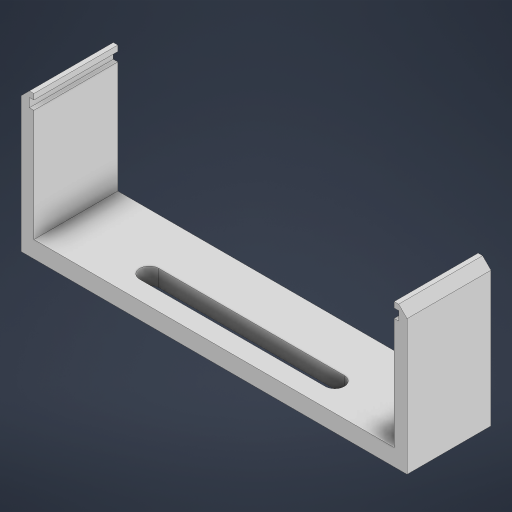
# Autodesk Inventor part: Discovery boar clamp
Saved by Autodesk Inventor 2023 (Build 270158000, 158)
## iProperties
Created: 2024-01-04
Part Number: Discovery boar clamp
Material: Generic
Document SubType Name: Modeling
Designer: nick_
Density: 1 g/cm^3
Appearance: Default
Author: nick_
Autodesk Inventor part; units mm, degrees
ref_plane "YZ Plane" through (0, 0, 0) normal (1, 0, 0) x (0, 1, 0)
ref_plane "XZ Plane" through (0, 0, 0) normal (0, 1, 0) x (-1, 0, 0)
ref_plane "XY Plane" through (0, 0, 0) normal (0, 0, 1) x (1, 0, 0)
sketch "Sketch1" plane through (0, 0, 0) normal (0, 0, 1) x (1, 0, 0)
  line L0 (0, 0) -> (-34.5, 0)
  line L1 (-34.5, 0) -> (-34.5, 25.6)
  line L2 (-34.5, 25.6) -> (-32.2, 25.6)
  line L3 (-32.2, 25.6) -> (-32.2, 24.6)
  line L4 (-32.2, 24.6) -> (-33, 24.6)
  line L5 (-33, 24.6) -> (-33, 23)
  line L6 (-33, 23) -> (-32.2, 23)
  line L7 (-32.2, 23) -> (-32.2, 3)
  line L8 (-32.2, 3) -> (0, 3)
  line L9 (0, 3) -> (0, 0)
  point P0 (-33, 23.8)
  point P1 (0, 1.5)
  dimension "d0" = 3
  dimension "d2" = 0.8
  dimension "d3" = 1
  dimension "d4" = 1.6
  dimension "d5" = 1.5
  dimension "d9" = 20
  dimension "d15" = 66
  constraints: 20 end point, 7 perpendicular, 2 midpoint, 1 horizontal, 1 parallel, 1 point on line, 1 vertical
  measures "d0" distance between parallel lines of L0 L8
  measures "d2" distance between parallel lines of L3 L5
  measures "d3" distance of L2.end L3.end
  measures "d4" distance of L4.end L5.end
  measures "d5" distance between parallel lines of L1 L5
  measures "d9" distance of L6.end L7.end
  measures "d15" diameter of L5 L9
extrude "Extrusion1" add sketch "Sketch1" along normal blind 15
mirror "Mirror1" about plane through (0, 0, 0) normal (1, 0, 0) of "Extrusion1"
sketch "Sketch2" plane through (-32.2, 3, 15) normal (0, 1, 0) x (1, 0, 0)
  line L0 (64.4, 15) -> (0, 15) construction
  line L1 (0, 15) -> (0, 0) construction
  line L2 (0, 0) -> (64.4, 0) construction
  line L3 (64.4, 15) -> (64.4, 0) construction
  line L4 (15.6221, 5) -> (48.7779, 5) construction
  line L5 (15.6221, 3.3) -> (48.7779, 3.3)
  line L6 (48.7779, 6.7) -> (15.6221, 6.7)
  arc A0 (15.6221, 6.7) -> (15.6221, 3.3) centre (15.6221, 5) ccw
  arc A1 (48.7779, 3.3) -> (48.7779, 6.7) centre (48.7779, 5) ccw
  point P0 (32.2, 15)
  point P1 (32.2, 5)
  point P2 (32.2, 15)
  dimension "d12" = 1.7
  constraints: 8 end point, 4 point on circle, 4 tangent, 2 centre point, 2 midpoint, 2 parallel, 1 vertical alignment
  measures "d12" radius of A0
extrude "Extrusion2" cut sketch "Sketch2" against normal through all
chamfer "Chamfer1" distance 1.5 angle 45 2 edges at (-34.5, 25.6, 7.5) (34.5, 25.6, 7.5)
body "Solid1"
